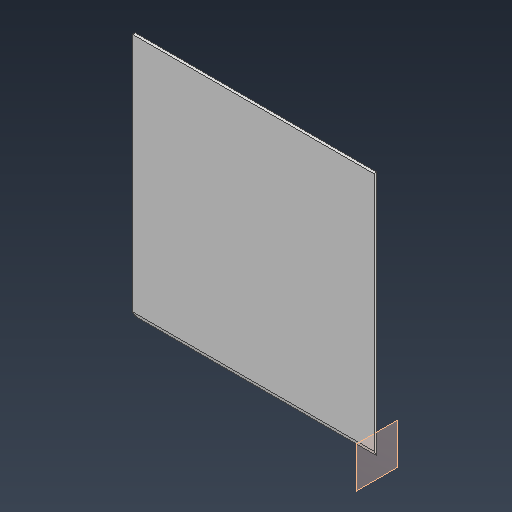
# Autodesk Inventor part: наклон
Saved by Autodesk Inventor 2025.2 (Build 292293000, 293)
## iProperties
Created: 2025-09-06
Part Number: наклон
Material: Типовые
Document SubType Name: Modeling
Designer: Trene
Density: 1 g/cm^3
Appearance: По умолчанию
Author: Trene
Autodesk Inventor part; units mm, degrees
ref_plane "YZ Plane" through (0, 0, 0) normal (1, 0, 0) x (0, 1, 0)
ref_plane "XZ Plane" through (0, 0, 0) normal (0, 1, 0) x (-1, 0, 0)
ref_plane "XY Plane" through (0, 0, 0) normal (0, 0, 1) x (1, 0, 0)
sketch "Эскиз1" plane through (0, 0, 0) normal (0, 0, 1) x (1, 0, 0)
  line L0 (0, 0) -> (130, 0)
  line L1 (130, 0) -> (130, 140)
  line L2 (130, 140) -> (0, 140)
  line L3 (0, 140) -> (0, 0)
  dimension "d0" = 130
  dimension "d1" = 140
  constraints: 8 end point, 2 parallel, 1 horizontal, 1 perpendicular
  measures "d0" distance of L2.end L1.end
  measures "d1" distance of L1.end L0.end
extrude "Выдавливание1" add sketch "Эскиз1" along normal blind 1.5
ref_plane "РабПлоскость1" through (130, 7.8819, 0) normal (1, 0, 0) x (0, 0, -1)
sketch "Эскиз3" plane through (130, 7.8819, 0) normal (1, 0, 0) x (0, 0, -1)
  line L0 (-1.5, 2.8482) -> (0, 0) projected
  line L1 (0, 0) -> (-1.5, 2.8482)
  line L2 (0, -7.8819) -> (0, 132.1181) projected
  line L3 (0, 132.1181) -> (-1.5, 132.1181) projected
  line L4 (-1.5, -7.8819) -> (-1.5, 132.1181) projected
  line L5 (0, -7.8819) -> (-1.5, -7.8819) projected
  point P0 (0, -7.8819)
  point P1 (0, 0)
  point P2 (-1.5, 2.8482)
  constraints: 2 end point, 1 collinear
extrude "Выдавливание3" cut sketch "Эскиз3" against normal through all contours L0 L2 L5 L4
